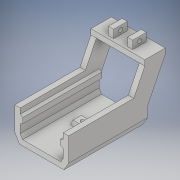
# Autodesk Inventor part: Ladeschlitten
Saved by Autodesk Inventor 2019 (Build 230136000, 136)
## iProperties
Created: 2022-03-16
Part Number: Ladeschlitten
Material: Generic
Document SubType Name: Modeling
Designer: Lukas
Density: 1 g/cm^3
Appearance: Default
Mass: 23.0436 g
Surface Area: 129.95 cm^2
Volume: 23.0436 cm^3
Author: Lukas
Autodesk Inventor part; units mm, degrees
ref_plane "YZ Plane" through (0, 0, 0) normal (1, 0, 0) x (0, 1, 0)
ref_plane "XZ Plane" through (0, 0, 0) normal (0, 1, 0) x (-1, 0, 0)
ref_plane "XY Plane" through (0, 0, 0) normal (0, 0, 1) x (1, 0, 0)
sketch "Sketch1" plane through (0, 0, 0) normal (0, 0, 1) x (1, 0, 0)
  line L0 (-14.0679, -10.6141) -> (14.0679, -10.6141)
  line L1 (14.0679, -10.6141) -> (15.8, -7.6141)
  line L2 (15.8, -7.6141) -> (15.8, -1.3141)
  line L3 (15.8, -1.3141) -> (13.8, -0.3141)
  line L4 (13.8, -0.3141) -> (13.8, 3.6859)
  line L5 (13.8, 3.6859) -> (15.8, 4.6859)
  line L6 (15.8, 4.6859) -> (15.8, 8.6859)
  line L7 (15.8, 8.6859) -> (19.8, 8.6859)
  line L8 (19.8, 8.6859) -> (19.8, -8.6859)
  line L9 (19.8, -8.6859) -> (16.3774, -14.6141)
  line L10 (16.3774, -14.6141) -> (-16.3774, -14.6141)
  line L11 (-16.3774, -14.6141) -> (-19.8, -8.6859)
  line L12 (-19.8, -8.6859) -> (-19.8, 8.6859)
  line L13 (-19.8, 8.6859) -> (-15.8, 8.6859)
  line L14 (-15.8, 8.6859) -> (-15.8, 4.6859)
  line L15 (-15.8, 4.6859) -> (-13.8, 3.6859)
  line L16 (-13.8, 3.6859) -> (-13.8, -0.3141)
  line L17 (-13.8, -0.3141) -> (-15.8, -1.3141)
  line L18 (-15.8, -1.3141) -> (-15.8, -7.6141)
  line L19 (-15.8, -7.6141) -> (-14.0679, -10.6141)
  point P0 (0, 0)
  point P1 (0, -14.6141)
  point P2 (-19.8, 0)
  dimension "d0" = 4
  dimension "d1" = 4
  dimension "d2" = 4
  dimension "d4" = 30
  dimension "d5" = 30
  dimension "d6" = 31.6
  dimension "d8" = 4
  dimension "d9" = 9.3
  dimension "d10" = 3
  dimension "d11" = 4
  dimension "d12" = 2
  dimension "d23" = 6
  dimension "d24" = 4
  constraints: 40 end point, 7 equal length, 6 point on line, 5 parallel, 4 perpendicular, 3 horizontal alignment, 2 midpoint, 1 horizontal, 1 vertical alignment
  measures "d0" distance between parallel lines of L0 L10
  measures "d1" distance between parallel lines of L9 L1
  measures "d2" distance between parallel lines of L19 L11
  measures "d4" angle of L11 L12
  measures "d5" angle of L8 L9
  measures "d6" distance between parallel lines of L6 L14
  measures "d8" distance of L12.end L13.end
  measures "d9" distance from line of L17.end L0
  measures "d10" distance from line of L0 L18.end
  measures "d11" distance of L15.end L16.end
  measures "d12" distance between parallel lines of L14 L16
  measures "d23" distance of L2.end L5.end
  measures "d24" distance of L13.end L14.end
extrude "Extrusion1" add sketch "Sketch1" along normal blind 58
sketch "Sketch2" plane through (-19.8, -8.6859, 0) normal (-1, 0, 0) x (0, 0, 1)
  line L0 (0, 0) -> (0, 17.3718) projected
  line L1 (0, 7.3718) -> (-13, 33.8718)
  line L2 (-13, 33.8718) -> (-13, 37.8718)
  line L3 (-13, 37.8718) -> (2, 37.8718)
  line L4 (0, 17.3718) -> (58, 17.3718) projected
  line L5 (58, 17.3718) -> (58, 0) projected
  line L6 (2, 37.8718) -> (2, 33.8718)
  line L7 (2, 33.8718) -> (10.0943, 17.3718)
  point P0 (0, 8.6859)
  point P1 (22.4242, 17.3718)
  point P2 (3, 17.3718)
  dimension "d17" = 4
  dimension "d41" = 2
  dimension "d42" = 10
  dimension "d43" = 15
  dimension "d44" = 20.5
  constraints: 10 end point, 4 point on line, 2 parallel, 1 horizontal alignment, 1 perpendicular, 1 vertical
  measures "d17" distance of L1.end L2.end
  measures "d41" distance from line of L3.end L0
  measures "d42" distance from line of L4 L1.start
  measures "d43" distance of L2.end L3.end
  measures "d44" distance between parallel lines of L4 L3
extrude "Extrusion2" add sketch "Sketch2" against normal up to surface (4 mm away)
mirror "Mirror1" about plane through (0, 0, 0) normal (1, 0, 0) of "Extrusion2"
sketch "Sketch3" plane through (15.8, 4.6859, 58) normal (-1, 0, 0) x (0, 0, 1)
  line L0 (-71, 20.5) -> (-71, 24.5) projected
  line L1 (-58, -6) -> (-71, 20.5) projected
  line L2 (-71, 24.5) -> (-71, 20.5)
  line L3 (-71, 20.5) -> (-56, 20.5)
  line L4 (-56, 24.5) -> (-71, 24.5) projected
  line L5 (-56, 24.5) -> (-56, 20.5)
  line L6 (-56, 24.5) -> (-71, 24.5)
  line L7 (-56, 20.5) -> (-56, 24.5) projected
  point P0 (-58, -4.6859)
  point P1 (-57, 21)
  constraints: 8 end point, 2 vertical, 1 parallel, 1 perpendicular, 3 other
extrude "Extrusion3" add sketch "Sketch3" along normal up to surface (31.6 mm away)
sketch "Sketch4" plane through (19.8, 29.1859, 2) normal (0, 1, 0) x (1, 0, 0)
  line L0 (-39.6, 15) -> (0, 15) projected
  line L1 (-28.7, 12) -> (-24.9, 12)
  line L2 (-24.9, 12) -> (-24.9, 2)
  line L3 (-24.9, 2) -> (-28.7, 2)
  line L4 (-28.7, 2) -> (-28.7, 12)
  line L5 (-14.7, 12) -> (-10.9, 12)
  line L6 (-10.9, 12) -> (-10.9, 2)
  line L7 (-10.9, 2) -> (-14.7, 2)
  line L8 (-14.7, 2) -> (-14.7, 12)
  line L9 (-19.8, 29.2) -> (-19.8, -70.2) projected
  dimension "d68" = 10.2
  dimension "d70" = 3
  dimension "d71" = 10
  dimension "d72" = 3.8
  dimension "d73" = 5.1
  constraints: 16 end point, 4 parallel, 2 horizontal, 2 horizontal alignment, 2 perpendicular, 2 point on line, 1 collinear
  measures "d68" distance between parallel lines of L8 L2
  measures "d70" distance between parallel lines of L0 L1
  measures "d71" distance of L3.end L1.start
  measures "d72" distance of L2.end L3.end
  measures "d73" distance between parallel lines of L9 L2
extrude "Extrusion6" add sketch "Sketch4" along normal blind 6
sketch "Sketch5" plane through (-8.9, 29.1859, 7) normal (-1, 0, 0) x (0, 1, 0)
  circle A0 centre (3, 12) radius 1.5
  line L0 (0, 17) -> (6, 17) projected
  line L1 (0, 7) -> (0, 17) projected
  point P0 (-26.2047, 8)
  dimension "d38" = 3
  dimension "d74" = 5
  dimension "d75" = 3
  constraints: 1 centre point
  measures "d38" diameter of A0
  measures "d74" distance from line of L0 A0.centre
  measures "d75" distance from line of L1 A0.centre
extrude "Extrusion5" cut sketch "Sketch5" against normal through all
sketch "Sketch6" plane through (-14.0679, -10.6141, 0) normal (0, 1, 0) x (1, 0, 0)
  line L0 (18.0679, -25) -> (10.0679, -25)
  line L1 (10.0679, -25) -> (10.0679, -31)
  line L2 (10.0679, -31) -> (18.0679, -31)
  line L3 (18.0679, -31) -> (18.0679, -25)
  line L4 (0, 0) -> (28.1359, 0) projected
  line L5 (28.1359, -58) -> (0, -58) projected
  circle A0 centre (14.0679, -28) radius 1.35
  point P0 (14.0679, 0)
  point P1 (14.0679, -25)
  point P2 (14.0679, 0)
  point P3 (18.0679, -28)
  point P4 (14.0679, -31)
  dimension "d53" = 6
  dimension "d54" = 8
  dimension "d55" = 30
  dimension "d56" = 2.7
  constraints: 8 end point, 4 midpoint, 2 parallel, 2 vertical alignment, 1 centre point, 1 horizontal, 1 horizontal alignment, 1 perpendicular
  measures "d53" distance of L2.end L0.start
  measures "d54" distance of L1.end L2.end
  measures "d55" distance from line of L5 A0.centre
  measures "d56" diameter of A0
extrude "Extrusion7" add sketch "Sketch6" along normal blind 4
chamfer "Chamfer1" distance 2 distance2 4 1 edges at (4, -10.6141, 28) measured on face at (4.5, -10.6141, 28)
chamfer "Chamfer2" distance 4 distance2 2 1 edges at (-4, -10.6141, 28) measured on face at (-4, -10.1141, 28)
chamfer "Chamfer3" distance 4 angle 45 3 edges at (-4.9999, -10.6141, 25) (0, -10.6141, 25) (4.9999, -10.6141, 25)
ref_plane "Work Plane1" through (0, 0, 0) normal (1, 0, 0) x (0, 1, 0)
equation "\"d4\" = d5"
equation "\"d73\" = 0.5 * d68"
body "Solid1"
